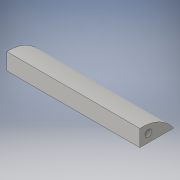
# Autodesk Inventor part: HingPart2
Saved by Autodesk Inventor 2016 (Build 200138000, 138)
## iProperties
Created: 2017-02-17
Part Number: HingPart2
Material: Generic
Document SubType Name: Modeling
Designer: RoboticsUser
Density: 1 g/cm^3
Appearance: Default
Author: RoboticsUser
Autodesk Inventor part; units mm, degrees
ref_plane "YZ Plane" through (0, 0, 0) normal (1, 0, 0) x (0, 1, 0)
ref_plane "XZ Plane" through (0, 0, 0) normal (0, 1, 0) x (-1, 0, 0)
ref_plane "XY Plane" through (0, 0, 0) normal (0, 0, 1) x (1, 0, 0)
sketch "Sketch1" plane through (0, 0, 0) normal (1, 0, 0) x (0, 1, 0)
  line L0 (0, 0) -> (0.0762, 0)
  line L1 (3.175, 5.5426) -> (3.175, 5.5426)
  line L2 (0, 0) -> (0.1524, 0)
  line L3 (0, 0) -> (0, 6.35)
  line L4 (0, 0) -> (0.1524, 0)
  line L5 (0, 6.35) -> (3.175, 6.35)
  arc A0 (0.1524, 0) -> (3.175, 6.35) centre (-4.1583, 5.9463) ccw
  dimension "d14" = 6.35
  dimension "d15" = 3.175
  constraints: 12 end point, 3 point on circle, 2 horizontal, 1 centre point, 1 midpoint, 1 parallel, 1 perpendicular, 1 point on line, 1 vertical
  measures "d14" distance of L0.start L3.end
  measures "d15" distance of L3.end L5.end
extrude "Extrusion2" add sketch "Sketch1" along normal blind 25.4
hole "Hole2" at (25.4, 1.6002, 4.7498) direction (-1, 0, 0) diameter 1.27 end through all
body "Solid2"
